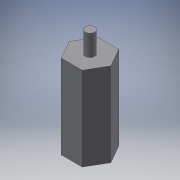
# Autodesk Inventor part: Part9
Saved by Autodesk Inventor 2016 (Build 200138000, 138)
## iProperties
Created: 2018-01-18
Part Number: Part9
Material: Generic
Document SubType Name: Modeling
Designer: student
Density: 1 g/cm^3
Appearance: Default
Author: student
Autodesk Inventor part; units mm, degrees
ref_plane "YZ Plane" through (0, 0, 0) normal (1, 0, 0) x (0, 1, 0)
ref_plane "XZ Plane" through (0, 0, 0) normal (0, 1, 0) x (-1, 0, 0)
ref_plane "XY Plane" through (0, 0, 0) normal (0, 0, 1) x (1, 0, 0)
sketch "Sketch1" plane through (0, 0, 0) normal (0, 1, 0) x (-1, 0, 0)
  circle A0 centre (130.4354, 61.1321) radius 1.4224
  point P0 (0, 0)
  dimension "d0" = 2.8448
  constraints: 1 centre point
  measures "d0" diameter of A0
extrude "Extrusion1" add sketch "Sketch1" along normal blind 6.35
sketch "Sketch2" plane through (-130.4354, 0, 61.1321) normal (0, -1, 0) x (1, 0, 0)
  circle A0 centre (0, 0) radius 1.4224 construction
  line L0 (3.1527, 5.5122) -> (6.35, 0.0258)
  line L1 (6.35, 0.0258) -> (3.1973, -5.4864)
  line L2 (3.1973, -5.4864) -> (-3.1527, -5.5122)
  line L3 (-3.1527, -5.5122) -> (-6.35, -0.0258)
  line L4 (-6.35, -0.0258) -> (-3.1973, 5.4864)
  line L5 (-3.1973, 5.4864) -> (3.1527, 5.5122)
  point P0 (130.4354, -61.1321)
  dimension "d3" = 6.35
  constraints: 12 end point, 1 coincident, 13 other
  measures "d3" horizontal distance of L4.end L0.start
extrude "Extrusion2" add sketch "Sketch2" along normal blind 25.4
sketch "Sketch3" plane through (-130.4354, -25.4, 61.1321) normal (0, -1, 0) x (1, 0, 0)
  circle A0 centre (0, 0) radius 1.4224 projected
  point P0 (130.4354, -61.1321)
extrude "Extrusion3" add sketch "Sketch3" along normal blind 6.35
body "Solid1"
